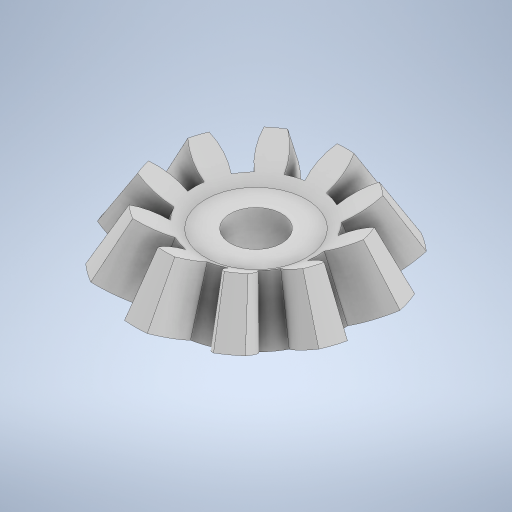
# Autodesk Inventor part: 베벨기어 002
Saved by Autodesk Inventor 2023 (Build 270158000, 158)
## iProperties
Created: 2022-06-18
Part Number: 베벨기어 002
Material: 일반
Document SubType Name: Modeling
Designer: fly01
Density: 1 g/cm^3
Appearance: 기본값
Author: fly01
Autodesk Inventor part; units mm, degrees
ref_plane "YZ Plane" through (0, 0, 0) normal (1, 0, 0) x (0, 1, 0)
ref_plane "XZ Plane" through (0, 0, 0) normal (0, 1, 0) x (-1, 0, 0)
ref_plane "XY Plane" through (0, 0, 0) normal (0, 0, 1) x (1, 0, 0)
sketch "스케치1" plane through (0, 0, 0) normal (0, 0, 1) x (1, 0, 0)
  line L0 (-10, 0) -> (10, 0) construction
  line L1 (0, 0) -> (0, 20) construction
  line L2 (0, 20) -> (10, 0) construction
  line L3 (0, 20) -> (11.7082, 1.0557)
  line L4 (0, 20) -> (7.8647, -1.3197) construction
  line L5 (7.8647, -1.3197) -> (11.7082, 1.0557)
  line L6 (7.8647, -1.3197) -> (7.0141, -1.8454)
  line L7 (7.0141, -1.8454) -> (3.9324, -1.8454)
  line L8 (3.9324, -1.8454) -> (3.9324, -3.5)
  line L9 (3.9324, -3.5) -> (0, -3.5)
  line L10 (8.7322, 5.871) -> (4.8959, 3.5)
  line L11 (4.8959, 3.5) -> (0, 3.5)
  line L12 (0, 3.5) -> (0, -3.5)
  dimension "d0" = 20
  dimension "d1" = 20
  dimension "d4" = 2
  dimension "d5" = 2.5
  dimension "d6" = 1
  dimension "d8" = 3
  dimension "d11" = 3.5
  dimension "d12" = 7
  constraints: 27 end point, 5 perpendicular, 4 point on line, 2 horizontal, 1 coincident, 1 collinear, 1 midpoint, 1 vertical
  measures "d0" distance of L0.start L0.end
  measures "d1" distance of L1.start L1.end
  measures "d4" distance from line of L3.end L2
  measures "d5" distance from line of L4.end L2
  measures "d6" distance of L4.end L6.end
  measures "d8" distance from line of L10.end L2
  measures "d11" distance between parallel lines of L0 L11
  measures "d12" distance between parallel lines of L11 L9
revolve "회전1" add sketch "스케치1" angle 360 about axis through (0, 3.5, 0) along (0, -1, 0)
ref_plane "작업 평면1" through (7.8647, -1.3197, 0) normal (-0.5257311, 0.8506508, 0) x (-0.8506508, -0.5257311, 0)
sketch "스케치3" plane through (7.8647, -1.3197, 0) normal (-0.5257311, 0.8506508, 0) x (-0.8506508, -0.5257311, 0)
  ellipse E0 centre (5.4413, 0) end of major axis (5.4413, 11.7082) minor radius 9.9596 construction
  line L0 (-4.5183, 0) -> (-2.5183, 0) construction
  line L1 (-2.5183, 0) -> (-0.0183, 0) construction
  ellipse E1 centre (5.4413, 0) end of major axis (5.4413, 9.6672) minor radius 7.9596 construction
  ellipse E2 centre (5.4413, 0) end of major axis (5.4413, 6.8965) minor radius 5.4596 (0.0479, 1.07) -> (0.0479, -1.07) ccw
  arc A0 (-4.2754, 2.57) -> (0.0479, 1.07) centre (0.3796, 9.0061) ccw
  arc A1 (0.0479, -1.07) -> (-4.2754, -2.57) centre (0.3796, -9.0061) ccw
  arc A2 (-4.2754, 2.57) -> (-4.2754, -2.57) centre (9.1992, 0) ccw
  line L2 (-4.2754, 2.57) -> (-5.6349, 2.57)
  line L3 (-5.6349, 2.57) -> (-5.6349, -2.57)
  line L4 (-5.6349, -2.57) -> (-4.2754, -2.57)
  point P0 (5.9964, 0)
  point P1 (-2.4126, 1.57)
  dimension "d21" = 2
  dimension "d22" = 2.5
  dimension "d23" = 1.57
  dimension "d26" = 0.5
  dimension "d27" = 1
  constraints: 10 end point, 8 point on circle, 3 centre point, 3 symmetric about line, 2 horizontal, 1 horizontal alignment, 1 perpendicular, 1 point on line, 1 vertical, 13 other
  measures "d21" distance of L0.start L0.end
  measures "d22" distance of L0.end L1.end
  measures "d23" distance from line of L0 point (-2.413, 1.57)
  measures "d26" vertical distance of point (-2.413, 1.57) A0.end
  measures "d27" vertical distance of point (-2.413, 1.57) L2.start
loft "로프트1" cut profiles "스케치3" section 2 point at (0, 20, 0)
pattern_circular "원형 패턴1" count 10 over 360 about axis through (0, 4.6855, 0) along (0, -1, 0) of "로프트1"
sketch "스케치4" plane through (0, 3.5, 0) normal (0, 1, 0) x (1, 0, 0)
  circle A0 centre (0, 0) radius 2.5
  dimension "d35" = 5
  constraints: 1 centre point, 1 coincident
  measures "d35" diameter of A0
extrude "돌출1" cut sketch "스케치4" against normal blind 30.75
